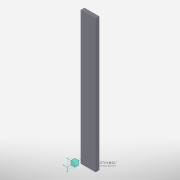
# Autodesk Inventor part: Y-servo-mount-bracket
Saved by Autodesk Inventor 2016 (Build 200138000, 138)
## iProperties
Created: 2015-05-21
Part Number: Y-servo-mount-bracket
Material: Generic
Document SubType Name: Modeling
Designer: as
Mass: 143.497 g
Surface Area: 374.149 cm^2
Volume: 143.497 cm^3
Density: 1 g/cm^3
Appearance: Default
Author: as
Autodesk Inventor part; units mm, degrees
ref_plane "YZ Plane" through (0, 0, 0) normal (1, 0, 0) x (0, 1, 0)
ref_plane "Work Plane1" through (-15, -10, 385) normal (0, 0, -1) x (0, 1, 0)
ref_plane "Work Plane2" through (-23.5, -10, 350) normal (0, 0, -1) x (0, 1, 0)
sketch "Sketch1" plane through (0, 0, 0) normal (0, 0, 1) x (1, 0, 0)
  line L0 (0, 0) -> (40, 0)
  line L1 (40, 0) -> (40, -10)
  line L2 (40, -10) -> (0, -10)
  line L3 (0, -10) -> (0, 0)
  dimension "d0" = 40
  dimension "d1" = 10
  constraints: 8 end point, 2 parallel, 1 horizontal, 1 perpendicular
  measures "d0" distance of L1.end L2.end
  measures "d1" distance of L0.end L1.end
extrude "Extrusion1" add sketch "Sketch1" along normal blind 360
sketch "Sketch2" plane through (0, -10, 0) normal (-1, 0, 0) x (0, 0, 1)
  point P0 (43, 5)
  point P1 (313, 5)
  point P2 (178, 5)
hole "Hole1" at (0, -5, 43) at (0, -5, 313) at (0, -5, 178) direction (1, 0, 0) diameter 3.242 depth 20 tip angle 120 thread size "M4x0.7" class "6H" standard "ISO Metric profile"
body "Solid1"
